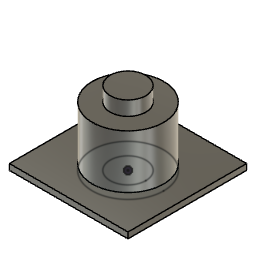
Arduino Pin v1 (Autodesk Fusion 360 design; units mm, degrees)
Autodesk Fusion 360 part; units mm, degrees
sketch "Skizze1" plane through (0, 0, 0) normal (0, 0, 1) x (1, 0, 0)
  circle A0 centre (0, 0) radius 3
  circle A1 centre (0, 0) radius 1.5
  dimension "d1" = 6
  dimension "d2" = 3
  constraint coincident A0.centre A1.centre
  measures "d1" diameter of A0
  measures "d2" diameter of A1
extrude "Extrusion1" add sketch "Skizze1" along normal blind 5
extrude "Extrusion2" add sketch "Skizze1" along normal blind 6.2 contours A1
sketch "Skizze2" plane through (0, 0, 0) normal (0, 0, 1) x (1, 0, 0)
  line L0 (-5, 5) -> (5, 5)
  line L1 (5, 5) -> (5, -5)
  line L2 (5, -5) -> (-5, -5)
  line L3 (-5, -5) -> (-5, 5)
  dimension "d9" = 10
  constraint horizontal L0
  constraint vertical L1
  constraint horizontal L2
  constraint vertical L3
  measures "d9" distance of L1 L3
extrude "Extrusion3" add sketch "Skizze2" along normal blind 0.5
equation "d5 = 5 mm + ( 0.12 * 10 ) * 1 mm"
